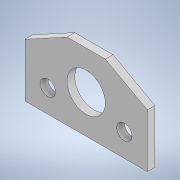
# Autodesk Inventor part: Assignment 4.3 - Positioning Stop
Saved by Autodesk Inventor 2022 (Build 260153000, 153)
## iProperties
Created: 2021-05-24
Part Number: Assignment 4.3 - Positioning Stop
Material: Generic
Document SubType Name: Modeling
Designer: Aaron
Density: 1 g/cm^3
Appearance: Default
Author: Aaron
Autodesk Inventor part; units mm, degrees
ref_plane "YZ Plane" through (0, 0, 0) normal (1, 0, 0) x (0, 1, 0)
ref_plane "XZ Plane" through (0, 0, 0) normal (0, 1, 0) x (-1, 0, 0)
ref_plane "XY Plane" through (0, 0, 0) normal (0, 0, 1) x (1, 0, 0)
sketch "Sketch1" plane through (0, 0, 0) normal (0, 0, 1) x (1, 0, 0)
  line L0 (0, 0) -> (101.6, 0)
  line L1 (101.6, 0) -> (101.6, 44.45)
  line L2 (0, 0) -> (0, 44.45)
  line L3 (34.925, 63.5) -> (66.675, 63.5)
  line L4 (66.675, 63.5) -> (101.6, 44.45)
  line L5 (34.925, 63.5) -> (0, 44.45)
  circle A0 centre (50.8, 31.75) radius 15.875
  circle A1 centre (19.05, 19.05) radius 6.35
  circle A2 centre (82.55, 19.05) radius 6.35
  dimension "d0" = 101.6
  dimension "d1" = 44.45
  dimension "d2" = 44.45
  dimension "d5" = 31.75
  dimension "d8" = 31.75
  dimension "d11" = 12.7
  dimension "d13" = 12.7
  constraints: 12 end point, 3 centre point, 1 horizontal, 1 perpendicular, 1 vertical
  measures "d0" distance of L0.start L0.end
  measures "d1" distance of L0.end L1.end
  measures "d2" distance of L0.start L2.end
  measures "d5" distance of L3.start L3.end
  measures "d8" diameter of A0
  measures "d11" diameter of A1
  measures "d13" diameter of A2
extrude "Extrusion1" add sketch "Sketch1" against normal blind 6.35
body "Solid1"
